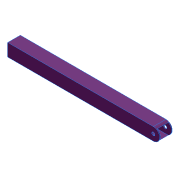
# Autodesk Inventor part: Shovel_Arm
Saved by Autodesk Inventor 2012 (Build 160160000, 160)
## iProperties
Created: 2013-01-29
Part Number: Shovel_Arm
Material: Aluminum-6061
Document SubType Name: Modeling
Designer: JesseK
Density: 2.71 g/cm^3
Mass: 122.398 g
Surface Area: 574.052 cm^2
Volume: 45.1652 cm^3
Author: JesseK
Autodesk Inventor part; units mm, degrees
ref_plane "YZ Plane" through (0, 0, 0) normal (1, 0, 0) x (0, 1, 0)
ref_plane "XZ Plane" through (0, 0, 0) normal (0, 1, 0) x (-1, 0, 0)
ref_plane "XY Plane" through (0, 0, 0) normal (0, 0, 1) x (1, 0, 0)
sketch "Sketch1" plane through (0, 0, 0) normal (0, 0, 1) x (1, 0, 0)
  line L0 (0, 0) -> (-304.8, 0)
  line L1 (-304.8, 0) -> (-304.8, 25.4)
  line L2 (-304.8, 25.4) -> (0, 25.4)
  line L3 (0, 25.4) -> (0, 0)
  dimension "d0" = 25.4
  dimension "d1" = 304.8
  constraints: 8 end point, 2 parallel, 1 horizontal, 1 perpendicular
  measures "d0" distance of L0.end L1.end
  measures "d1" distance of L1.end L2.end
extrude "Extrusion1" add sketch "Sketch1" along normal blind 25.4
shell "Shell1" thickness 1.5875 removed faces 2 at (0, 16.9333, 8.4667) at (-304.8, 8.4667, 8.4667)
sketch "Sketch2" plane through (0, 0, 25.4) normal (0, 0, 1) x (1, 0, 0)
  line L0 (0, 0) -> (-304.8, 0) projected
  line L1 (0, 25.4) -> (0, 0) projected
  circle A0 centre (-12.7, 12.7) radius 3.175
  dimension "d5" = 12.7
  dimension "d6" = 12.7
  dimension "d7" = 6.35
  constraints: 1 centre point
  measures "d5" distance from line of L0 A0.centre
  measures "d6" distance from line of L1 A0.centre
  measures "d7" diameter of A0
extrude "Extrusion2" cut sketch "Sketch2" against normal through all
fillet "Fillet1" radius 12.7 2 edges at (0, 25.4, 12.7) (0, 0, 12.7)
body "Solid1"
